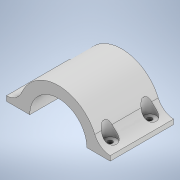
# Autodesk Inventor part: mocowanie silnika górne
Saved by Autodesk Inventor 2021 (Build 250183000, 183)
## iProperties
Created: 2021-06-29
Part Number: mocowanie silnika górne
Material: Generic
Document SubType Name: Modeling
Designer: Łukasz
Density: 1 g/cm^3
Appearance: Default
Author: Łukasz
Autodesk Inventor part; units mm, degrees
ref_plane "YZ Plane" through (0, 0, 0) normal (1, 0, 0) x (0, 1, 0)
ref_plane "XZ Plane" through (0, 0, 0) normal (0, 1, 0) x (-1, 0, 0)
sketch "Sketch1" plane through (0, 0, 0) normal (0, 0, 1) x (1, 0, 0)
  arc A0 (18, 0) -> (-18, 0) centre (0, 0) ccw
  arc A1 (24.8193, 3) -> (-24.8193, 3) centre (0, 0) ccw
  line L0 (-25, 0) -> (-32.75, 0)
  line L1 (-32.75, 0) -> (-32.75, 3)
  line L2 (-32.75, 3) -> (-24.8193, 3)
  line L3 (25, 0) -> (32.75, 0)
  line L4 (32.75, 0) -> (32.75, 3)
  line L5 (32.75, 3) -> (24.8193, 3)
  line L6 (-25, 0) -> (-18, 0)
  line L7 (25, 0) -> (18, 0)
  dimension "d0" = 36
  dimension "d1" = 50
  dimension "d2" = 7.75
  dimension "d3" = 3
  dimension "d4" = 7.75
  dimension "d5" = 3
  constraints: 16 end point, 5 point on line, 4 point on circle, 2 centre point, 2 coincident, 2 horizontal, 2 perpendicular, 1 collinear
  measures "d0" diameter of A0
  measures "d1" diameter of A1
  measures "d2" distance of L0.start L0.end
  measures "d3" distance of L0.end L1.end
  measures "d4" distance of L3.start L3.end
  measures "d5" distance of L3.end L4.end
extrude "Extrusion1" add sketch "Sketch1" along normal blind 40
fillet "Fillet1" radius 11 2 edges at (24.8193, 3, 20) (-24.8193, 3, 20)
sketch "Sketch2" plane through (-32.75, 0, 0) normal (0, -1, 0) x (1, 0, 0)
  circle A0 centre (7.5, 7.5) radius 1.5
  line L0 (-36, 0) -> (0, 0)
  line L1 (0, 0) -> (0, 0)
  circle A1 centre (58, 7.5) radius 1.5
  circle A2 centre (7.5, 32.5) radius 1.5
  circle A3 centre (58, 32.5) radius 1.5
  line L2 (0, 0) -> (0, 40) projected
  line L3 (0, 0) -> (14.75, 0) projected
  point P0 (32.75, 0)
  point P1 (-18, 0)
  dimension "d13" = 3
  dimension "d14" = 7.5
  dimension "d15" = 7.5
  dimension "d16" = 50.5
  dimension "d17" = 25
  dimension "d18" = 0
  dimension "d19" = 0
  constraints: 4 centre point, 4 end point, 1 horizontal, 1 vertical, 6 other
  measures "d13" diameter of A0
  measures "d14" distance from line of L0 A0.centre
  measures "d15" distance from line of L1 A0.centre
  measures "d16" distance of A0.centre A1.centre
  measures "d17" distance of A0.centre A2.centre
  measures "d18" distance between parallel lines of L2 L1
  measures "d19" distance between parallel lines of L3 L0
extrude "Extrusion2" cut sketch "Sketch2" against normal blind 40
ref_plane "Work Plane1" through (-32.75, 3, 0) normal (0, -1, 0) x (1, 0, 0)
sketch "Sketch3" plane through (-32.75, 3, 0) normal (0, -1, 0) x (1, 0, 0)
  circle A0 centre (7.5, 7.5) radius 1.5 projected
  circle A1 centre (7.5, 7.5) radius 4
  circle A2 centre (7.5, 32.5) radius 1.5 projected
  circle A3 centre (7.5, 32.5) radius 4
  circle A4 centre (58, 32.5) radius 1.5 projected
  circle A5 centre (58, 32.5) radius 4
  circle A6 centre (58, 7.5) radius 4
  point P0 (32.75, 0)
  dimension "d23" = 8
  dimension "d24" = 8
  dimension "d25" = 8
  dimension "d26" = 8
  constraints: 4 centre point, 3 coincident
  measures "d23" diameter of A1
  measures "d24" diameter of A3
  measures "d25" diameter of A5
  measures "d26" diameter of A6
extrude "Extrusion3" cut sketch "Sketch3" against normal blind 10 contours A0 | A1 | A2 | A3 | A4 | A5 | A6
body "Solid1"
